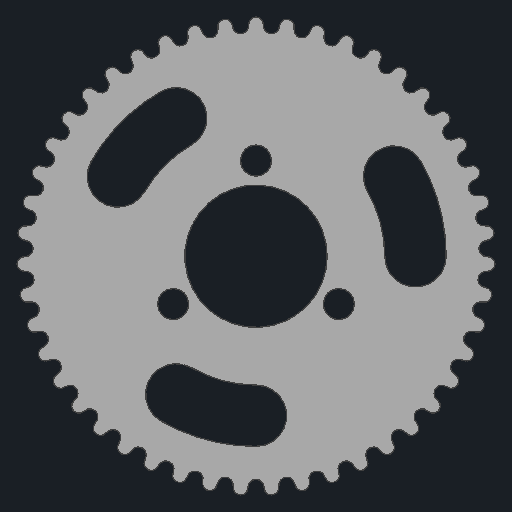
# Autodesk Inventor part: SprocketMDEOOSKY-25H-47T
Saved by Autodesk Inventor 2025.2 (Build 292293000, 293)
## iProperties
Created: 2025-10-11
Part Number: SprocketMDEOOSKY-25H-47T
Material: Generic
Document SubType Name: Sheet Metal
Designer: valer
Density: 1 g/cm^3
Sheet Metal Rule: Default_mm
Appearance: Default
Author: valer
Autodesk Inventor part; units mm, degrees
ref_plane "YZ Plane" through (0, 0, 0) normal (1, 0, 0) x (0, 1, 0)
ref_plane "XZ Plane" through (0, 0, 0) normal (0, 1, 0) x (-1, 0, 0)
ref_plane "XY Plane" through (0, 0, 0) normal (0, 0, 1) x (1, 0, 0)
sketch "Base" plane through (0, 0, 0) normal (0, 0, 1) x (1, 0, 0)
  circle A0 centre (0, 0) radius 48.75
  circle A1 centre (0, 0) radius 14.5
  circle A2 centre (0, 0) radius 19.5 construction
  circle A3 centre (0, 19.5) radius 3.175
  line L0 (-68.25, 0) -> (68.25, 0) construction
  line L1 (0, -68.25) -> (0, 68.25) construction
  circle A4 centre (-16.8875, -9.75) radius 3.175
  circle A5 centre (16.8875, -9.75) radius 3.175
  circle A6 centre (0, 0) radius 32.5 construction
  arc A7 (-16.25, 28.1458) -> (-28.1458, 16.25) centre (0, 0) ccw construction
  arc A8 (-19.375, 33.5585) -> (-33.5585, 19.375) centre (0, 0) ccw
  arc A9 (-13.125, 22.7332) -> (-22.7332, 13.125) centre (0, 0) ccw
  arc A10 (-13.125, 22.7332) -> (-19.375, 33.5585) centre (-16.25, 28.1458) ccw
  arc A11 (-33.5585, 19.375) -> (-22.7332, 13.125) centre (-28.1458, 16.25) ccw
  line L2 (-16.25, 28.1458) -> (0, 0) construction
  line L3 (-28.1458, 16.25) -> (0, 0) construction
  arc A12 (-19.375, -33.5585) -> (0, -38.75) centre (0, 0) ccw
  arc A13 (-13.125, -22.7332) -> (-19.375, -33.5585) centre (-16.25, -28.1458) ccw
  arc A14 (-13.125, -22.7332) -> (0, -26.25) centre (0, 0) ccw
  arc A15 (0, -38.75) -> (0, -26.25) centre (0, -32.5) ccw
  arc A16 (38.75, 0) -> (33.5585, 19.375) centre (0, 0) ccw
  arc A17 (26.25, 0) -> (38.75, 0) centre (32.5, 0) ccw
  arc A18 (26.25, 0) -> (22.7332, 13.125) centre (0, 0) ccw
  arc A19 (33.5585, 19.375) -> (22.7332, 13.125) centre (28.1458, 16.25) ccw
  line L4 (0, 0) -> (-3.2561, 48.6411) construction
  circle A20 centre (-3.1454, 46.9866) radius 1.6583
  line L5 (0, 0) -> (3.2561, 48.6411) construction
  line L6 (0, 0) -> (0, 48.75) construction
  circle A21 centre (0, 45.6977) radius 3.0523 construction
  circle A22 centre (3.1454, 46.9866) radius 1.6583
  circle A23 centre (0, 47.2517) radius 1.4983
  circle A24 centre (-9.38, 46.1481) radius 1.6583
  circle A25 centre (-6.298, 46.8301) radius 1.4983
  circle A26 centre (-3.1454, 46.9866) radius 1.6583
  circle A27 centre (-15.4473, 44.4861) radius 1.6583
  circle A28 centre (-12.4837, 45.5728) radius 1.4983
  circle A29 centre (-9.38, 46.1481) radius 1.6583
  circle A30 centre (-21.2389, 42.0303) radius 1.6583
  circle A31 centre (-18.4466, 43.5023) radius 1.4983
  circle A32 centre (-15.4473, 44.4861) radius 1.6583
  circle A33 centre (-26.6514, 38.8244) radius 1.6583
  circle A34 centre (-24.0803, 40.6554) radius 1.4983
  circle A35 centre (-21.2389, 42.0303) radius 1.6583
  circle A36 centre (-31.5884, 34.9257) radius 1.6583
  circle A37 centre (-29.2842, 37.0831) radius 1.4983
  circle A38 centre (-26.6514, 38.8244) radius 1.6583
  circle A39 centre (-35.9617, 30.4037) radius 1.6583
  circle A40 centre (-33.9657, 32.849) radius 1.4983
  circle A41 centre (-31.5884, 34.9257) radius 1.6583
  circle A42 centre (-39.6933, 25.3392) radius 1.6583
  circle A43 centre (-38.0409, 28.0288) radius 1.4983
  circle A44 centre (-35.9617, 30.4037) radius 1.6583
  circle A45 centre (-42.7165, 19.8226) radius 1.6583
  circle A46 centre (-41.4374, 22.7083) radius 1.4983
  circle A47 centre (-39.6933, 25.3392) radius 1.6583
  circle A48 centre (-44.9774, 13.9521) radius 1.6583
  circle A49 centre (-44.0944, 16.9826) radius 1.4983
  circle A50 centre (-42.7165, 19.8226) radius 1.6583
  circle A51 centre (-46.4358, 7.8327) radius 1.6583
  circle A52 centre (-45.9645, 10.9539) radius 1.4983
  circle A53 centre (-44.9774, 13.9521) radius 1.6583
  circle A54 centre (-47.0655, 1.5736) radius 1.6583
  circle A55 centre (-47.0144, 4.7297) radius 1.4983
  circle A56 centre (-46.4358, 7.8327) radius 1.6583
  circle A57 centre (-46.8552, -4.7137) radius 1.6583
  circle A58 centre (-47.2253, -1.5789) radius 1.4983
  circle A59 centre (-47.0655, 1.5736) radius 1.6583
  circle A60 centre (-45.8089, -10.9168) radius 1.6583
  circle A61 centre (-46.5935, -7.8593) radius 1.4983
  circle A62 centre (-46.8552, -4.7137) radius 1.6583
  circle A63 centre (-43.9451, -16.9251) radius 1.6583
  circle A64 centre (-45.1302, -13.9995) radius 1.4983
  circle A65 centre (-45.8089, -10.9168) radius 1.6583
  circle A66 centre (-41.2971, -22.6314) radius 1.6583
  circle A67 centre (-42.8616, -19.8899) radius 1.4983
  circle A68 centre (-43.9451, -16.9251) radius 1.6583
  circle A69 centre (-37.9122, -27.9339) radius 1.6583
  circle A70 centre (-39.8281, -25.4253) radius 1.4983
  circle A71 centre (-41.2971, -22.6314) radius 1.6583
  circle A72 centre (-33.8507, -32.7378) radius 1.6583
  circle A73 centre (-36.0839, -30.507) radius 1.4983
  circle A74 centre (-37.9122, -27.9339) radius 1.6583
  circle A75 centre (-29.1851, -36.9576) radius 1.6583
  circle A76 centre (-31.6957, -35.0443) radius 1.4983
  circle A77 centre (-33.8507, -32.7378) radius 1.6583
  circle A78 centre (-23.9987, -40.5178) radius 1.6583
  circle A79 centre (-26.742, -38.9563) radius 1.4983
  circle A80 centre (-29.1851, -36.9576) radius 1.6583
  circle A81 centre (-18.3841, -43.355) radius 1.6583
  circle A82 centre (-21.311, -42.173) radius 1.4983
  circle A83 centre (-23.9987, -40.5178) radius 1.6583
  circle A84 centre (-12.4414, -45.4185) radius 1.6583
  circle A85 centre (-15.4997, -44.6372) radius 1.4983
  circle A86 centre (-18.3841, -43.355) radius 1.6583
  circle A87 centre (-6.2767, -46.6716) radius 1.6583
  circle A88 centre (-9.4119, -46.3049) radius 1.4983
  circle A89 centre (-12.4414, -45.4185) radius 1.6583
  circle A90 centre (0, -47.0918) radius 1.6583
  circle A91 centre (-3.1561, -47.1462) radius 1.4983
  circle A92 centre (-6.2767, -46.6716) radius 1.6583
  circle A93 centre (6.2767, -46.6716) radius 1.6583
  circle A94 centre (3.1561, -47.1462) radius 1.4983
  circle A95 centre (0, -47.0918) radius 1.6583
  circle A96 centre (12.4414, -45.4185) radius 1.6583
  circle A97 centre (9.4119, -46.3049) radius 1.4983
  circle A98 centre (6.2767, -46.6716) radius 1.6583
  circle A99 centre (18.3841, -43.355) radius 1.6583
  circle A100 centre (15.4997, -44.6372) radius 1.4983
  circle A101 centre (12.4414, -45.4185) radius 1.6583
  circle A102 centre (23.9987, -40.5178) radius 1.6583
  circle A103 centre (21.311, -42.173) radius 1.4983
  circle A104 centre (18.3841, -43.355) radius 1.6583
  circle A105 centre (29.1851, -36.9576) radius 1.6583
  circle A106 centre (26.742, -38.9563) radius 1.4983
  circle A107 centre (23.9987, -40.5178) radius 1.6583
  circle A108 centre (33.8507, -32.7378) radius 1.6583
  circle A109 centre (31.6957, -35.0443) radius 1.4983
  circle A110 centre (29.1851, -36.9576) radius 1.6583
  circle A111 centre (37.9122, -27.9339) radius 1.6583
  circle A112 centre (36.0839, -30.507) radius 1.4983
  circle A113 centre (33.8507, -32.7378) radius 1.6583
  circle A114 centre (41.2971, -22.6314) radius 1.6583
  circle A115 centre (39.8281, -25.4253) radius 1.4983
  circle A116 centre (37.9122, -27.9339) radius 1.6583
  circle A117 centre (43.9451, -16.9251) radius 1.6583
  circle A118 centre (42.8616, -19.8899) radius 1.4983
  circle A119 centre (41.2971, -22.6314) radius 1.6583
  circle A120 centre (45.8089, -10.9168) radius 1.6583
  circle A121 centre (45.1302, -13.9995) radius 1.4983
  circle A122 centre (43.9451, -16.9251) radius 1.6583
  circle A123 centre (46.8552, -4.7137) radius 1.6583
  circle A124 centre (46.5935, -7.8593) radius 1.4983
  circle A125 centre (45.8089, -10.9168) radius 1.6583
  circle A126 centre (47.0655, 1.5736) radius 1.6583
  circle A127 centre (47.2253, -1.5789) radius 1.4983
  circle A128 centre (46.8552, -4.7137) radius 1.6583
  circle A129 centre (46.4358, 7.8327) radius 1.6583
  circle A130 centre (47.0144, 4.7297) radius 1.4983
  circle A131 centre (47.0655, 1.5736) radius 1.6583
  circle A132 centre (44.9774, 13.9521) radius 1.6583
  circle A133 centre (45.9645, 10.9539) radius 1.4983
  circle A134 centre (46.4358, 7.8327) radius 1.6583
  circle A135 centre (42.7165, 19.8226) radius 1.6583
  circle A136 centre (44.0944, 16.9826) radius 1.4983
  circle A137 centre (44.9774, 13.9521) radius 1.6583
  circle A138 centre (39.6933, 25.3392) radius 1.6583
  circle A139 centre (41.4374, 22.7083) radius 1.4983
  circle A140 centre (42.7165, 19.8226) radius 1.6583
  circle A141 centre (35.9617, 30.4037) radius 1.6583
  circle A142 centre (38.0409, 28.0288) radius 1.4983
  circle A143 centre (39.6933, 25.3392) radius 1.6583
  circle A144 centre (31.5884, 34.9257) radius 1.6583
  circle A145 centre (33.9657, 32.849) radius 1.4983
  circle A146 centre (35.9617, 30.4037) radius 1.6583
  circle A147 centre (26.6514, 38.8244) radius 1.6583
  circle A148 centre (29.2842, 37.0831) radius 1.4983
  circle A149 centre (31.5884, 34.9257) radius 1.6583
  circle A150 centre (21.2389, 42.0303) radius 1.6583
  circle A151 centre (24.0803, 40.6554) radius 1.4983
  circle A152 centre (26.6514, 38.8244) radius 1.6583
  circle A153 centre (15.4473, 44.4861) radius 1.6583
  circle A154 centre (18.4466, 43.5023) radius 1.4983
  circle A155 centre (21.2389, 42.0303) radius 1.6583
  circle A156 centre (9.38, 46.1481) radius 1.6583
  circle A157 centre (12.4837, 45.5728) radius 1.4983
  circle A158 centre (15.4473, 44.4861) radius 1.6583
  circle A159 centre (3.1454, 46.9866) radius 1.6583
  circle A160 centre (6.298, 46.8301) radius 1.4983
  circle A161 centre (9.38, 46.1481) radius 1.6583
  point P0 (4.8016, 46.9044)
  point P1 (1.493, 47.1259)
  point P2 (-1.493, 47.1259)
  point P3 (-4.8016, 46.9044)
  point P4 (-7.7609, 46.5064)
  point P5 (-11.0105, 45.8459)
  point P6 (-13.8904, 45.057)
  point P7 (-17.0229, 43.9693)
  point P8 (-19.772, 42.8036)
  point P9 (-22.7316, 41.308)
  point P10 (-25.3007, 39.7863)
  point P11 (-28.0346, 37.9096)
  point P12 (-30.378, 36.0591)
  point P13 (-32.8373, 33.8347)
  point P14 (-34.9131, 31.6883)
  point P15 (-37.054, 29.1561)
  point P16 (-38.8252, 26.7521)
  point P17 (-40.6095, 23.9571)
  point P18 (-42.0445, 21.3386)
  point P19 (-43.4404, 18.3306)
  point P20 (-44.5135, 15.5442)
  point P21 (-45.496, 12.377)
  point P22 (-46.1882, 9.4724)
  point P23 (-46.7398, 6.2026)
  point P24 (-47.0386, 3.2316)
  point P25 (-47.1494, -0.0826)
  point P26 (-47.0497, -3.0669)
  point P27 (-46.7177, -6.3662)
  point P28 (-46.2211, -9.3106)
  point P29 (-45.4524, -12.5363)
  point P30 (-44.5677, -15.3882)
  point P31 (-43.3759, -18.4826)
  point P32 (-42.119, -21.1912)
  point P33 (-40.5254, -24.0992)
  point P34 (-38.9187, -26.616)
  point P35 (-36.9517, -29.2856)
  point P36 (-35.0239, -31.5659)
  point P37 (-32.7186, -33.9495)
  point P38 (-30.504, -35.9525)
  point P39 (-27.9016, -38.0076)
  point P40 (-25.4399, -39.6975)
  point P41 (-22.5868, -41.3874)
  point P42 (-19.9217, -42.7341)
  point P43 (-16.8688, -44.0286)
  point P44 (-14.0481, -45.0081)
  point P45 (-10.8499, -45.8842)
  point P46 (-7.9237, -46.4789)
  point P47 (-4.6373, -46.9209)
  point P48 (-1.658, -47.1204)
  point P49 (1.658, -47.1204)
  point P50 (4.6373, -46.9209)
  point P51 (7.9237, -46.4789)
  point P52 (10.8499, -45.8842)
  point P53 (14.0481, -45.0081)
  point P54 (16.8688, -44.0286)
  point P55 (19.9217, -42.7341)
  point P56 (22.5868, -41.3874)
  point P57 (25.4399, -39.6975)
  point P58 (27.9016, -38.0076)
  point P59 (30.504, -35.9525)
  point P60 (32.7186, -33.9495)
  point P61 (35.0239, -31.5659)
  point P62 (36.9517, -29.2856)
  point P63 (38.9187, -26.616)
  point P64 (40.5254, -24.0992)
  point P65 (42.119, -21.1912)
  point P66 (43.3759, -18.4826)
  point P67 (44.5677, -15.3882)
  point P68 (45.4524, -12.5363)
  point P69 (46.2211, -9.3106)
  point P70 (46.7177, -6.3662)
  point P71 (47.0497, -3.0669)
  point P72 (47.1494, -0.0826)
  point P73 (47.0386, 3.2316)
  point P74 (46.7398, 6.2026)
  point P75 (46.1882, 9.4724)
  point P76 (45.496, 12.377)
  point P77 (44.5135, 15.5442)
  point P78 (43.4404, 18.3306)
  point P79 (42.0445, 21.3386)
  point P80 (40.6095, 23.9571)
  point P81 (38.8252, 26.7521)
  point P82 (37.054, 29.1561)
  point P83 (34.9131, 31.6883)
  point P84 (32.8373, 33.8347)
  point P85 (30.378, 36.0591)
  point P86 (28.0346, 37.9096)
  point P87 (25.3007, 39.7863)
  point P88 (22.7316, 41.308)
  point P89 (19.772, 42.8036)
  point P90 (17.0229, 43.9693)
  point P91 (13.8904, 45.057)
  point P92 (11.0105, 45.8459)
  point P93 (7.7609, 46.5064)
  dimension "d2" = 39
  dimension "d8" = 65
  dimension "d0" = 97.5
  dimension "d1" = 29
  dimension "d3" = 6.35
  dimension "d6" = 360
  dimension "d9" = 30
  dimension "d10" = 30
  dimension "d13" = 360
  dimension "d15" = 6.25
  dimension "d17" = 3.3165
  dimension "d22" = 360
  measures "d0" diameter of A0
  measures "d1" diameter of A1
  measures "d3" diameter of A3
  measures "d9" angle of L1 L2
  measures "d10" angle of L0 L3
  measures "d15" radius of A10
  measures "d17" diameter of A20
extrude "Plate1" add sketch "Base" along normal blind 2.7 contours A133 | A127 | A130 | A94 | A126 A127 A123 A124 A120 A121 A117 A118 A114 A115 A111 A112 A108 A109 A105 A106 A102 A103 A99 A100 A96 A97 A93 A94 A90 A91 A87 A88 A84 A85 A81 A82 A78 A79 A75 A76 A72 A73 A69 A70 A66 A67 A63 A64 A60 A61 A57 A58 A54 A55 A51 A52 A48 A49 A45 A46 A42 A43 A39 A40 A36 A37 A33 A34 A30 A31 A27 A28 A24 A25 A20 A23 A22 A160 A156 A157 A153 A154 A150 A151 A147 A148 A144 A145 A141 A142 A138 A139 A135 A136 A132 A133 A129 A130 | A124 | A121 | A136 | A118 | A139 | A115 | A142 | A112 | A145 | A109 | A148 | A106 | A151 | A103 | A154 | A100 | A157 | A97 | A160 | A23 | A91 | A25 | A88 | A28 | A85 | A31 | A82 | A34 | A79 | A37 | A76 | A40 | A73 | A43 | A70 | A46 | A67 | A49 | A64 | A52 | A61 | A55 | A58
equation "\"d10\" = d9"
equation "\"BendRadius\" = Thickness"
equation "\"BendReliefWidth\" = Thickness"
equation "\"BendReliefDepth\" = 0.5 * Thickness"
equation "\"CornerReliefSize\" = 4 * Thickness"
equation "\"MinimumRemnant\" = 2 * Thickness"
equation "\"TransitionRadius\" = BendRadius"
equation "\"JacobiRadiusSize\" = BendRadius"
equation "\"GapSize\" = Thickness"
equation "\"Thickness\" = 2.7"
body "Solid1"
